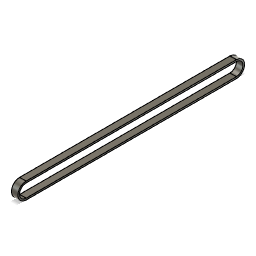
Ремень под мотор v5 (Autodesk Fusion 360 design; units mm, degrees)
Autodesk Fusion 360 part; units mm, degrees
sketch "Sketch1" plane through (0, 0, 0) normal (1, 0, 0) x (0, 0, -1)
  line L0 (0.0109, -6.1) -> (194.9888, -6.1)
  line L1 (195, 6.1) -> (0, 6.1)
  arc A0 (0, 6.1) -> (0.0109, -6.1) centre (0, 0) ccw
  arc A1 (194.9888, -6.1) -> (195, 6.1) centre (194.9888, 0) ccw
  line L2 (-0.0034, -7.6) -> (194.9888, -7.6)
  arc A2 (194.9888, -7.6) -> (195.0014, 7.6) centre (194.9888, 0) ccw
  line L3 (195.0014, 7.6) -> (0, 7.6)
  arc A3 (0, 7.6) -> (-0.0034, -7.6) centre (0, 0) ccw
  line L4 (0, 0) -> (194.9888, 0)
  dimension "d5" = 1.5
  dimension "d8" = 6.1
  dimension "d9" = 6.1
  dimension "d10" = 12.2
  dimension "d11" = 195
  constraint coincident A0.centre A3.centre
  constraint tangent L0 A1
  constraint tangent L1 A0
  constraint horizontal L4
  constraint coincident A1.centre A2.centre
  measures "d8" radius of A0
  measures "d9" radius of A1
  measures "d10" distance of L0 L1
  measures "d11" distance of L1.end L1.start
extrude "Extrude1" add sketch "Sketch1" along normal blind 6
sketch "Sketch2" plane through (0, 0, 0) normal (-1, 0, 0) x (0, 0, 1)
  arc A0 (-195, 6.1) -> (-194.9888, -6.1) centre (-194.9888, 0) ccw
  line L0 (-195, 6.1) -> (0, 6.1)
  arc A1 (-0.0109, -6.1) -> (0, 6.1) centre (0, 0) ccw
  line L1 (-0.0109, -6.1) -> (-194.9888, -6.1)
  arc A2 (0.0034, -7.6) -> (0, 7.6) centre (0, 0) ccw
  line L2 (0, 7.6) -> (-195.0014, 7.6)
  arc A3 (-195.0014, 7.6) -> (-194.9888, -7.6) centre (-194.9888, 0) ccw
  line L3 (-194.9888, -7.6) -> (0.0034, -7.6)
  line L4 (-0.004, 3.865) -> (-0.004, -8.2436)
  constraint vertical L4
sketch "Sketch3" plane through (0, 0, 0) normal (-1, 0, 0) x (0, 0, 1)
  arc A0 (-0.5, 5.9) -> (0.6, 5.9) centre (0.05, 5.95) ccw
